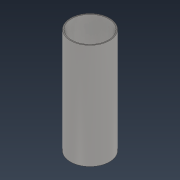
# Autodesk Inventor part: Cylinder
Saved by Autodesk Inventor 2022 (Build 260153000, 153)
## iProperties
Created: 2023-04-12
Part Number: Cylinder
Material: Stainless Steel, Austenitic
Document SubType Name: Modeling
Designer: wikto
Density: 8 g/cm^3
Appearance: Semi-Polished
Author: wikto
Autodesk Inventor part; units mm, degrees
ref_plane "YZ Plane" through (0, 0, 0) normal (1, 0, 0) x (0, 1, 0)
ref_plane "XZ Plane" through (0, 0, 0) normal (0, 1, 0) x (-1, 0, 0)
ref_plane "XY Plane" through (0, 0, 0) normal (0, 0, 1) x (1, 0, 0)
sketch "Sketch1" plane through (0, 0, 0) normal (0, 1, 0) x (-1, 0, 0)
  circle A0 centre (0, 0) radius 50
  circle A1 centre (0, 0) radius 53
  dimension "d0" = 100
  dimension "d1" = 3
  constraints: 2 centre point, 2 coincident
  measures "d0" diameter of A0
  measures "d1" radial gap between concentric circles of A0 A1
extrude "Extrusion1" add sketch "Sketch1" along normal blind 285
body "Solid1"
